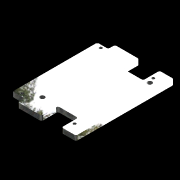
# Autodesk Inventor part: 3d_LM - chapa
Saved by Autodesk Inventor 2018.3 (Build 223284000, 284)
## iProperties
Created: 2025-11-25
Part Number: 3d_LM - chapa
Material: Aluminium 6061-T6
Document SubType Name: Modeling
Designer: mbs18
Density: 2.7 g/cm^3
Appearance: N/A - Machined Aluminium
Mass: 19.8311 g
Surface Area: 53.684 cm^2
Volume: 7.34487 cm^3
Author: mbs18
Comments: DIN-ISO-2768-fH
Autodesk Inventor part; units mm, degrees
ref_plane "YZ Plane" through (0, 0, 0) normal (1, 0, 0) x (0, 1, 0)
ref_plane "XZ Plane" through (0, 0, 0) normal (0, 1, 0) x (-1, 0, 0)
ref_plane "XY Plane" through (0, 0, 0) normal (0, 0, 1) x (1, 0, 0)
sketch "Sketch1" plane through (0, 0, 0) normal (0, 0, 1) x (1, 0, 0)
  line L0 (10.66, -31.5) -> (10.66, -19.9) construction
  line L1 (10.66, -31.5) -> (20, -31.5) construction
  line L2 (20, -31.5) -> (20, 31.5) construction
  line L3 (10.66, 31.5) -> (20, 31.5) construction
  line L4 (10.66, 19.9) -> (10.66, 31.5) construction
  arc A0 (9.66, 18.9) -> (10.66, 19.9) centre (9.66, 19.9) ccw construction
  line L5 (2.06, 18.9) -> (9.66, 18.9) construction
  arc A1 (1.06, 19.9) -> (2.06, 18.9) centre (2.06, 19.9) ccw construction
  line L6 (1.06, 31.5) -> (1.06, 19.9) construction
  line L7 (-20, 31.5) -> (1.06, 31.5) construction
  line L8 (-20, 31.5) -> (-20, -31.5) construction
  line L9 (-20, -31.5) -> (1.06, -31.5) construction
  line L10 (1.06, -19.9) -> (1.06, -31.5) construction
  arc A2 (2.06, -18.9) -> (1.06, -19.9) centre (2.06, -19.9) ccw construction
  line L11 (9.66, -18.9) -> (2.06, -18.9) construction
  arc A3 (10.66, -19.9) -> (9.66, -18.9) centre (9.66, -19.9) ccw construction
  line L12 (17.245, 17.9) -> (-18.765, 17.9) construction
  line L13 (17.245, -17.9) -> (17.245, 17.9) construction
  line L14 (-18.765, -17.9) -> (17.245, -17.9) construction
  line L15 (-18.765, 17.9) -> (-18.765, -17.9) construction
  circle A4 centre (0.9382, -13.2582) radius 1 construction
  circle A5 centre (-15.16, -21.5982) radius 1 construction
  circle A6 centre (-15.16, 21.6018) radius 1 construction
  circle A7 centre (13.64, 21.6018) radius 1 construction
  line L16 (10.84, 17.8518) -> (1.765, 17.8518)
  arc A8 (0.765, 18.8518) -> (1.765, 17.8518) centre (1.765, 18.8518) ccw
  line L17 (0.765, 26.467) -> (0.765, 18.8518)
  arc A9 (0.765, 26.467) -> (-0.06, 26.9018) centre (-0.06, 25.9018) ccw
  line L18 (-0.06, 26.9018) -> (-12.68, 26.9018)
  line L19 (-12.68, 26.9018) -> (-12.68, 24.2118)
  arc A10 (-13.68, 23.2118) -> (-12.68, 24.2118) centre (-13.68, 24.2118) ccw
  line L20 (-17.78, 23.2118) -> (-13.68, 23.2118)
  arc A11 (-18.78, 24.2118) -> (-17.78, 23.2118) centre (-17.78, 24.2118) ccw
  line L21 (-18.78, 26.9018) -> (-18.78, 24.2118)
  line L22 (-18.78, 26.9018) -> (-20.66, 26.9018)
  line L23 (-20.66, 26.9018) -> (-20.66, -26.8982)
  line L24 (-18.55, -26.8982) -> (-20.66, -26.8982)
  line L25 (-18.55, -26.8982) -> (-18.55, -24.2182)
  arc A12 (-17.55, -23.2182) -> (-18.55, -24.2182) centre (-17.55, -24.2182) ccw
  line L26 (-13.38, -23.2182) -> (-17.55, -23.2182)
  arc A13 (-12.38, -24.2182) -> (-13.38, -23.2182) centre (-13.38, -24.2182) ccw
  line L27 (-12.38, -26.8982) -> (-12.38, -24.2182)
  line L28 (-0.06, -26.8982) -> (-12.38, -26.8982)
  arc A14 (-0.06, -26.8982) -> (0.77, -26.4559) centre (-0.06, -25.8982) ccw
  line L29 (0.77, -26.4559) -> (0.77, -18.8482)
  arc A15 (1.77, -17.8482) -> (0.77, -18.8482) centre (1.77, -18.8482) ccw
  line L30 (1.77, -17.8482) -> (10.84, -17.8482)
  arc A16 (11.84, -18.8482) -> (10.84, -17.8482) centre (10.84, -18.8482) ccw
  line L31 (11.84, -18.8482) -> (11.84, -25.8982)
  arc A17 (11.84, -25.8982) -> (12.84, -26.8982) centre (12.84, -25.8982) ccw
  line L32 (17.74, -26.8982) -> (12.84, -26.8982)
  line L33 (17.74, -26.8982) -> (17.74, 26.9018)
  line L34 (17.74, 26.9018) -> (12.84, 26.9018)
  arc A18 (12.84, 26.9018) -> (11.84, 25.9018) centre (12.84, 25.9018) ccw
  line L35 (11.84, 25.9018) -> (11.84, 18.8518)
  arc A19 (10.84, 17.8518) -> (11.84, 18.8518) centre (10.84, 18.8518) ccw
  circle A20 centre (-15.16, 21.6018) radius 1
  circle A21 centre (-15.16, -21.5982) radius 1
  circle A22 centre (13.64, -21.5982) radius 1
  circle A23 centre (13.64, 21.6018) radius 1
  line L36 (-20.66, 0.0018) -> (17.74, 0.0018) construction
  line L37 (-1.46, 0.0018) -> (-1.46, -26.8982) construction
  line L38 (-20, 0) -> (20, 0) construction
  point P0 (-20.66, -26.8983)
  point P1 (17.64, 32.8018)
  dimension "d2" = 40
  dimension "d3" = 63
  constraints: 78 end point, 32 point on circle, 24 centre point, 5 midpoint, 1 perpendicular, 1 point on line
  measures "d2" distance between parallel lines of L2 L8
  measures "d3" distance between parallel lines of L9 L7
extrude "Extrusion1" add sketch "Sketch1" against normal blind 2.7 contours A19 L35 A18 L34 L33 L32 A17 L31 A16 L30 A15 L29 A14 L28 L27 A13 L26 A12 L25 L24 L23 L22 L21 A11 L20 A10 L19 L18 A9 L17 A8 L16 | A20 | A21 | A22 | A23
hole "Hole1" at (-15.16, -21.5982, 0) at (-15.16, 21.6018, 0) at (13.64, 21.6018, 0) at (13.64, -21.5982, 0) at (13.64, 21.6018, 0) at (-15.16, 21.6018, 0) at (-15.16, -21.5982, 0) direction (0, 0, -1) diameter 1.567 depth 2.5 thread size "M2x0.4" class "6H" standard "ISO Metric profile"
sketch "Sketch2" plane through (0, 0, -2.7) normal (0, 0, -1) x (-1, 0, 0)
  circle A0 centre (-14.8923, 18.4994) radius 1.6002 projected
  circle A1 centre (7.7497, -17.8506) radius 1.6002 projected
  line L0 (-14.8923, 18.4994) -> (7.7497, 18.4994)
  line L1 (7.7497, 18.4994) -> (7.7497, -17.8506)
  line L2 (7.7497, -17.8506) -> (-14.8923, -17.8506)
  line L3 (-14.8923, -17.8506) -> (-14.8923, 18.4994)
  constraints: 8 end point, 2 coincident, 2 parallel, 1 horizontal, 1 perpendicular
hole "Hole2" at (-7.7497, -17.8506, -2.7) at (14.8923, 18.4994, -2.7) direction (0, 0, 1) diameter 2.459 end through all thread size "M3x0.5" class "6H" standard "ISO Metric profile"
sketch "Sketch4" plane through (0, 0, 0) normal (0, 0, 1) x (1, 0, 0)
  line L0 (-20.66, 26.9018) -> (-18.78, 26.9018) projected
  line L1 (-17.78, 23.2118) -> (-20.66, 23.2118)
  line L2 (-20.66, 23.2118) -> (-20.66, 26.9018)
  line L3 (-20.66, 26.9018) -> (-17.78, 26.9018)
  line L4 (-17.78, 26.9018) -> (-17.78, 23.2118)
  line L5 (-18.55, -26.8982) -> (-20.66, -26.8982) projected
  line L6 (-17.55, -23.2182) -> (-20.66, -23.2182)
  line L7 (-20.66, -23.2182) -> (-20.66, -26.8982)
  line L8 (-20.66, -26.8982) -> (-17.55, -26.8982)
  line L9 (-17.55, -26.8982) -> (-17.55, -23.2182)
  point P0 (0, 0)
  constraints: 16 end point, 4 parallel, 2 horizontal, 2 perpendicular
extrude "Extrusion4" cut sketch "Sketch4" against normal blind 10
sketch "Sketch5" plane through (-20.66, -23.2182, 0) normal (-1, 0, 0) x (0, 0, 1)
  line L0 (0, 46.43) -> (-2.7, 46.43) projected
  line L1 (-2.7, 0) -> (-2.7, 46.43) projected
  line L2 (-2.7, 0) -> (0, 0) projected
  line L3 (0, 46.43) -> (0, 0) projected
  point P0 (0, 23.2182)
extrude "Extrusion5" cut sketch "Sketch5" against normal blind 2
sketch "Sketch6" plane through (17.74, -26.8982, 0) normal (1, 0, 0) x (0, 0, -1)
  line L0 (0, 0) -> (0, 53.8) projected
  line L1 (0, 0) -> (2.7, 0) projected
  line L2 (2.7, 53.8) -> (2.7, 0) projected
  line L3 (0, 53.8) -> (2.7, 53.8) projected
  point P0 (0, 26.8982)
extrude "Extrusion6" add sketch "Sketch6" along normal blind 2
sketch "Sketch7" plane through (0, 0, -2.7) normal (0, 0, -1) x (-1, 0, 0)
  arc A0 (-0.77, -26.4559) -> (0.06, -26.8982) centre (0.06, -25.8982) ccw projected
  line L0 (-0.77, -26.4559) -> (0.06, -26.4559)
  line L1 (0.06, -26.4559) -> (0.06, -26.8982)
  line L2 (0.06, -26.8982) -> (-0.77, -26.8982)
  line L3 (-0.77, -26.8982) -> (-0.77, -26.4559)
  arc A1 (0.06, 26.9018) -> (-0.765, 26.467) centre (0.06, 25.9018) ccw projected
  line L4 (0.06, 26.9018) -> (-0.765, 26.9018)
  line L5 (-0.765, 26.9018) -> (-0.765, 26.467)
  line L6 (-0.765, 26.467) -> (0.06, 26.467)
  line L7 (0.06, 26.467) -> (0.06, 26.9018)
  point P0 (0, 0)
  constraints: 16 end point, 4 parallel, 2 horizontal, 2 perpendicular
extrude "Extrusion7" add sketch "Sketch7" against normal up to surface (2.7 mm away)
fillet "Fillet3" radius 1 6 edges at (-12.38, -26.8982, -1.35) (19.74, -26.8982, -1.35) (19.74, 26.9018, -1.35) (-12.68, 26.9018, -1.35) (0.765, 26.9018, -1.35) (0.77, -26.8982, -1.35)
body "Solid1"
